Autodesk Inventor part; units mm, degrees
(part 2 of 3)
sketch "CylindricalPathOption2" plane through (0, 0, 0) normal (0, 1, 0) x (1, 0, 0)
  circle A0 centre (-38.1, 345.52) radius 3.175 projected
  circle A1 centre (-88.9, 345.52) radius 3.175 projected
  line L0 (-139.469, 321.04) -> (-139.469, 70.086)
  line L1 (-139.469, 321.04) -> (-144.509, 321.04)
  line L2 (-38.1, 459.82) -> (-101.369, 459.82)
  circle A2 centre (-101.369, 459.82) radius 3.175
  line L3 (-101.369, 459.82) -> (-139.469, 459.82)
  circle A3 centre (-139.469, 459.82) radius 3.175
  line L4 (-139.469, 459.82) -> (-139.469, 357.4623)
  circle A4 centre (-134.429, 321.04) radius 1.016
  line L5 (-139.469, 459.82) -> (-139.469, 321.04)
  line L6 (-139.469, 321.04) -> (-134.429, 321.04)
  circle A5 centre (-139.469, 321.04) radius 3.175
  circle A6 centre (-144.509, 321.04) radius 1.016
  line L7 (-139.469, 459.82) -> (-239.869, 459.82)
  circle A7 centre (-239.869, 459.82) radius 3.175
  circle A8 centre (-134.429, 70.086) radius 1.016
  circle A9 centre (-144.509, 70.086) radius 1.016
  circle A10 centre (-139.469, 70.086) radius 3.175
  line L8 (-139.469, 70.086) -> (-139.469, -143.414)
  circle A11 centre (-134.429, -143.414) radius 1.016
  circle A12 centre (-144.509, -143.414) radius 1.016
  circle A13 centre (-139.469, -143.414) radius 3.175
  line L9 (-38.1, 459.82) -> (-26.0664, 459.82)
  line L10 (-26.0664, 459.82) -> (-26.0664, 471.8536)
  circle A14 centre (-22.5281, 468.3152) radius 1.016
  circle A15 centre (-29.6048, 475.3919) radius 1.016
  circle A16 centre (-26.0664, 471.8536) radius 3.175
  line L11 (-38.1, 459.82) -> (-101.369, 459.82) projected
  point P0 (0, 0)
  point P1 (-38.1, 345.52)
  point P2 (-88.9, 345.52)
  point P3 (-134.429, 70.086)
  dimension "d423" = 12.0335
  dimension "d424" = 12.0335
  dimension "d425" = 6.35
  dimension "d426" = 2.032
  dimension "d427" = 2.032
  dimension "d428" = 63.269
  dimension "d429" = 6.35
  dimension "d430" = 38.1
  dimension "d431" = 100.4
  dimension "d432" = 138.78
  dimension "d433" = 250.954
  dimension "d434" = 213.5
  dimension "d435" = 5.04
  dimension "d436" = 5.04
  dimension "d437" = 2.032
  dimension "d438" = 2.032
  dimension "d439" = 6.35
  dimension "d440" = 5.04
  dimension "d441" = 5.04
  dimension "d442" = 2.032
  dimension "d443" = 2.032
  dimension "d444" = 6.35
  dimension "d445" = 5.04
  dimension "d446" = 5.04
  dimension "d447" = 2.032
  dimension "d448" = 2.032
  dimension "d449" = 6.35
  constraints: 22 end point, 15 centre point, 12 coincident, 2 horizontal, 2 point on line, 1 perpendicular, 1 vertical
  measures "d423" distance of L2.start L9.end
  measures "d424" distance of L9.end L10.end
  measures "d425" diameter of A16
  measures "d426" diameter of A15
  measures "d427" diameter of A14
  measures "d428" distance of L2.start L2.end
  measures "d429" diameter of A2
  measures "d430" distance of L3.start L3.end
  measures "d431" distance of L7.start L7.end
  measures "d432" distance of L5.start L1.start
  measures "d433" distance of L1.start L0.end
  measures "d434" distance of L0.end L8.end
  measures "d435" distance of L1.start L6.end
  measures "d436" distance of L1.start L1.end
  measures "d437" diameter of A6
  measures "d438" diameter of A4
  measures "d439" diameter of A5
  measures "d440" distance of point (-139.469, 70.086) point (-134.429, 70.086)
  measures "d441" distance of point (-139.469, 70.086) point (-144.509, 70.086)
  measures "d442" diameter of A9
  measures "d443" diameter of A8
  measures "d444" diameter of A10
  measures "d445" distance of point (-139.469, -143.414) point (-134.429, -143.414)
  measures "d446" distance of point (-139.469, -143.414) point (-144.509, -143.414)
  measures "d447" diameter of A12
  measures "d448" diameter of A11
  measures "d449" diameter of A13
sketch "CylindricalPathOption3" plane through (0, 0, 0) normal (0, 1, 0) x (1, 0, 0)
  circle A0 centre (-38.1, 80.7174) radius 3.175
  line L0 (-38.1, 320.3874) -> (-43.104, 320.3874)
  line L1 (-38.1, 320.3874) -> (-33.096, 320.3874)
  circle A1 centre (-33.096, 320.3874) radius 1.016
  circle A2 centre (-43.104, 320.3874) radius 1.016
  circle A3 centre (-38.1, 320.3874) radius 3.175
  line L2 (-38.1, 282.2874) -> (-43.104, 282.2874)
  circle A4 centre (-43.104, 282.2874) radius 1.016
  line L3 (-38.1, 282.2874) -> (-38.1, 320.3874)
  line L4 (-38.1, 282.2874) -> (-33.096, 282.2874)
  circle A5 centre (-38.1, 282.2874) radius 3.175
  circle A6 centre (-33.096, 282.2874) radius 1.016
  line L5 (-38.1, 244.1874) -> (-43.104, 244.1874)
  line L6 (-38.1, 244.1874) -> (-33.096, 244.1874)
  circle A7 centre (-33.096, 244.1874) radius 1.016
  circle A8 centre (-43.104, 244.1874) radius 1.016
  circle A9 centre (-38.1, 244.1874) radius 3.175
  line L7 (-38.1, 244.1874) -> (-38.1, 282.2874)
  line L8 (-38.1, 413.5374) -> (-33.096, 413.5374)
  line L9 (-38.1, 413.5374) -> (-38.1, 591.1064)
  circle A10 centre (-33.096, 413.5374) radius 1.016
  circle A11 centre (-33.096, 409.7056) radius 1.016
  circle A12 centre (-33.096, 80.7174) radius 1.016
  circle A13 centre (-43.104, 80.7174) radius 1.016
  circle A14 centre (-38.1, 80.7174) radius 3.175
  line L10 (-38.1, 68.0174) -> (-38.1, 80.7174)
  line L11 (0, 68.0174) -> (-38.1, 68.0174)
  line L12 (-38.1, 80.7174) -> (-33.096, 80.7174)
  line L13 (-38.1, 80.7174) -> (-43.104, 80.7174)
  line L14 (-38.1, 80.7174) -> (-38.1, 156.9174)
  line L15 (-38.1, 156.9174) -> (-43.104, 156.9174)
  line L16 (-38.1, 156.9174) -> (-33.096, 156.9174)
  circle A15 centre (-33.096, 156.9174) radius 1.016
  circle A16 centre (-43.104, 156.9174) radius 1.016
  circle A17 centre (-38.1, 156.9174) radius 3.175
  line L17 (-38.1, 156.9174) -> (-38.1, 174.0274)
  circle A18 centre (-33.096, 174.0274) radius 1.016
  line L18 (-38.1, 174.0274) -> (-33.096, 174.0274)
  line L19 (-38.1, 174.0274) -> (-38.1, 244.1874)
  line L20 (-38.1, 174.0274) -> (-43.104, 174.0274)
  circle A19 centre (-38.1, 174.0274) radius 3.175
  circle A20 centre (-43.104, 174.0274) radius 1.016
  line L21 (-38.1, 320.3874) -> (-38.1, 413.5374)
  line L22 (-38.1, 591.1064) -> (-38.1, 629.2064)
  circle A21 centre (-38.1, 591.1064) radius 3.175
  circle A22 centre (-33.096, 591.1064) radius 1.016
  line L23 (-38.1, 629.2064) -> (-43.104, 629.2064)
  line L24 (-38.1, 629.2064) -> (-33.096, 629.2064)
  circle A23 centre (-33.096, 629.2064) radius 1.016
  circle A24 centre (-43.104, 629.2064) radius 1.016
  circle A25 centre (-38.1, 629.2064) radius 3.175
  line L25 (-38.1, 591.1064) -> (-33.096, 591.1064)
  line L26 (-38.1, 591.1064) -> (-43.104, 591.1064)
  circle A26 centre (-43.104, 591.1064) radius 1.016
  line L27 (-38.1, 413.5374) -> (-38.1, 409.7056)
  circle A27 centre (-38.1, 409.7056) radius 3.175
  circle A28 centre (-38.1, 413.5374) radius 3.175
  line L28 (-38.1, 413.5374) -> (-43.104, 413.5374)
  circle A29 centre (-43.104, 409.7056) radius 1.016
  circle A30 centre (-43.104, 413.5374) radius 1.016
  circle A31 centre (-83.896, 413.5374) radius 1.016
  line L29 (-38.1, 413.5374) -> (-88.9, 413.5374)
  circle A32 centre (-88.9, 413.5374) radius 3.175
  circle A33 centre (-84.547, 90.1756) radius 1.016
  line L30 (-38.1, 629.2064) -> (-38.1, 729.6064)
  line L31 (-38.1, 729.6064) -> (-43.104, 729.6064)
  line L32 (-38.1, 729.6064) -> (-33.096, 729.6064)
  circle A34 centre (-43.104, 729.6064) radius 1.016
  circle A35 centre (-33.096, 729.6064) radius 1.016
  circle A36 centre (-38.1, 729.6064) radius 3.175
  line L33 (-63.5, 742.3174) -> (-38.1, 742.3174)
  line L34 (-38.1, 729.6064) -> (-38.1, 742.3174)
  line L35 (-38.1, 413.5374) -> (-38.1, 451.6374)
  line L36 (-14.6636, 459.2391) -> (108.4085, 459.2391) construction
  line L37 (108.4085, 459.2391) -> (108.4085, 436.8992) construction
  line L38 (108.4085, 436.8992) -> (-14.6636, 436.8992) construction
  line L39 (-14.6636, 436.8992) -> (-14.6636, 459.2391) construction
  line L40 (-38.1, 413.5374) -> (-38.1, 527.8374)
  line L41 (-38.1, 527.8374) -> (-101.369, 527.8374)
  line L42 (-139.469, 527.8374) -> (-239.869, 527.8374)
  circle A37 centre (-239.869, 527.8374) radius 3.175
  circle A38 centre (-139.469, 527.8374) radius 3.175
  circle A39 centre (-101.369, 527.8374) radius 3.175
  line L43 (-101.369, 527.8374) -> (-139.469, 527.8374)
  line L44 (-139.469, 389.0574) -> (-144.509, 389.0574)
  line L45 (-139.469, 527.8374) -> (-139.469, 389.0574)
  circle A40 centre (-144.509, 389.0574) radius 1.016
  line L46 (-139.469, 389.0574) -> (-134.429, 389.0574)
  circle A41 centre (-139.469, 389.0574) radius 3.175
  circle A42 centre (-134.429, 389.0574) radius 1.016
  line L47 (-139.469, 389.0574) -> (-139.469, 138.1034)
  line L48 (-139.469, 527.8374) -> (-139.469, 425.4797)
  circle A43 centre (-139.469, 138.1034) radius 3.175
  circle A44 centre (-144.509, 138.1034) radius 1.016
  circle A45 centre (-134.429, -75.3966) radius 1.016
  line L49 (-139.469, 138.1034) -> (-139.469, -75.3966)
  circle A46 centre (-144.509, -75.3966) radius 1.016
  circle A47 centre (-139.469, -75.3966) radius 3.175
  circle A48 centre (-134.429, 138.1034) radius 1.016
  line L50 (-38.1, 527.8374) -> (-101.369, 527.8374)
  line L51 (-38.1, 527.8374) -> (-26.0664, 527.8374)
  line L52 (-26.0664, 527.8374) -> (-26.0664, 539.871)
  circle A49 centre (-29.6048, 543.4093) radius 1.016
  circle A50 centre (-22.5281, 536.3326) radius 1.016
  circle A51 centre (-26.0664, 539.871) radius 3.175
  circle A52 centre (-26.0664, 539.871) radius 3.175 projected
  circle A53 centre (-29.6048, 543.4093) radius 1.0125 projected
  circle A54 centre (-22.5281, 536.3326) radius 1.0125 projected
  point P0 (0, 0)
  point P1 (0, 68.0174)
  point P2 (-38.1, 409.7056)
  dimension "d450" = 38.1
  dimension "d451" = 12.7
  dimension "d452" = 76.2
  dimension "d453" = 17.11
  dimension "d454" = 70.16
  dimension "d455" = 38.1
  dimension "d456" = 38.1
  dimension "d457" = 93.15
  dimension "d458" = 177.569
  dimension "d459" = 38.1
  dimension "d460" = 100.4
  dimension "d461" = 5.004
  dimension "d462" = 5.004
  dimension "d463" = 2.032
  dimension "d464" = 2.032
  dimension "d465" = 6.35
  dimension "d466" = 5.004
  dimension "d467" = 5.004
  dimension "d468" = 2.032
  dimension "d469" = 2.032
  dimension "d470" = 6.35
  dimension "d471" = 5.004
  dimension "d472" = 5.004
  dimension "d473" = 2.032
  dimension "d474" = 2.032
  dimension "d475" = 6.35
  dimension "d476" = 5.004
  dimension "d477" = 5.004
  dimension "d478" = 2.032
  dimension "d479" = 2.032
  dimension "d480" = 6.35
  dimension "d481" = 5.004
  dimension "d482" = 5.004
  dimension "d483" = 2.032
  dimension "d484" = 2.032
  dimension "d485" = 6.35
  dimension "d486" = 5.004
  dimension "d487" = 5.004
  dimension "d488" = 2.032
  dimension "d489" = 2.032
  dimension "d490" = 6.35
  dimension "d491" = 5.004
  dimension "d492" = 5.004
  dimension "d493" = 2.032
  dimension "d494" = 2.032
  dimension "d495" = 6.35
  dimension "d496" = 5.004
  dimension "d497" = 5.004
  dimension "d498" = 2.032
  dimension "d499" = 2.032
  dimension "d500" = 6.35
  dimension "d501" = 5.004
  dimension "d502" = 5.004
  dimension "d503" = 2.032
  dimension "d504" = 2.032
  dimension "d505" = 6.35
  dimension "d506" = 5.004
  dimension "d507" = 5.004
  dimension "d508" = 2.032
  dimension "d509" = 2.032
  dimension "d510" = 6.35
  dimension "d511" = 50.8
  dimension "d512" = 2.032
  dimension "d513" = 2.032
  constraints: 98 end point, 52 centre point, 42 coincident, 24 horizontal, 11 point on line, 3 vertical, 2 perpendicular, 2 other
  measures "d450" distance of L11.start L10.start
  measures "d451" distance of L10.start L13.start
  measures "d452" distance of L13.start L14.end
  measures "d453" distance of L14.end L19.start
  measures "d454" distance of L19.start L7.start
  measures "d455" distance of L7.start L7.end
  measures "d456" distance of L7.end L3.end
  measures "d457" distance of L3.end L9.start
  measures "d458" distance of L9.start L9.end
  measures "d459" distance of L9.end L22.end
  measures "d460" distance of L22.end L30.end
  measures "d461" distance of L13.start L12.end
  measures "d462" distance of L13.start L13.end
  measures "d463" diameter of A12
  measures "d464" diameter of A13
  measures "d465" diameter of A14
  measures "d466" distance of L15.start L16.end
  measures "d467" distance of L15.start L15.end
  measures "d468" diameter of A15
  measures "d469" diameter of A16
  measures "d470" diameter of A17
  measures "d471" distance of L20.start L18.end
  measures "d472" distance of L20.start L20.end
  measures "d473" diameter of A18
  measures "d474" diameter of A20
  measures "d475" diameter of A19
  measures "d476" distance of L5.start L6.end
  measures "d477" distance of L5.start L5.end
  measures "d478" diameter of A7
  measures "d479" diameter of A8
  measures "d480" diameter of A9
  measures "d481" distance of L2.start L4.end
  measures "d482" distance of L2.start L2.end
  measures "d483" diameter of A6
  measures "d484" diameter of A4
  measures "d485" diameter of A5
  measures "d486" distance of L1.start L1.end
  measures "d487" distance of L1.start L0.end
  measures "d488" diameter of A1
  measures "d489" diameter of A2
  measures "d490" diameter of A3
  measures "d491" distance of L29.start L8.end
  measures "d492" distance of L29.start L28.end
  measures "d493" diameter of A10
  measures "d494" diameter of A30
  measures "d495" diameter of A28
  measures "d496" distance of L26.start L25.end
  measures "d497" distance of L26.start L26.end
  measures "d498" diameter of A22
  measures "d499" diameter of A26
  measures "d500" diameter of A21
  measures "d501" distance of L23.start L24.end
  measures "d502" distance of L23.start L23.end
  measures "d503" diameter of A23
  measures "d504" diameter of A24
  measures "d505" diameter of A25
  measures "d506" distance of L31.start L32.end
  measures "d507" distance of L31.start L31.end
  measures "d508" diameter of A35
  measures "d509" diameter of A34
  measures "d510" diameter of A36
  measures "d511" distance of L29.start L29.end
  measures "d512" diameter of A31
  measures "d513" diameter of A33
sketch "CylindricalPathOption3_CTaslmHoles" plane through (0, 0, 0) normal (0, 1, 0) x (1, 0, 0)
  circle A0 centre (-139.469, 389.0574) radius 3.175 projected
  line L0 (-139.469, 389.0574) -> (-139.469, 156.3064)
  line L1 (-139.469, 156.3064) -> (-139.469, -53.4156)
  circle A1 centre (-144.509, 389.0574) radius 1.016 projected
  line L2 (-139.469, 389.0574) -> (-144.509, 389.0574) projected
  line L3 (-139.469, 389.0574) -> (-134.429, 389.0574) projected
  circle A2 centre (-134.429, 389.0574) radius 1.016 projected
  line L4 (-139.469, 389.0574) -> (-139.469, 138.1034) projected
  line L5 (-139.469, 527.8374) -> (-139.469, 389.0574) projected
  circle A3 centre (-139.469, 156.3064) radius 3.175
  circle A4 centre (-139.469, -53.4156) radius 3.175
  line L6 (-139.469, 156.3064) -> (-144.473, 156.3064)
  line L7 (-139.469, 156.3064) -> (-134.465, 156.3064)
  circle A5 centre (-144.473, 156.3064) radius 1.016
  circle A6 centre (-134.465, 156.3064) radius 1.016
  circle A7 centre (-139.469, -53.4156) radius 3.175
  line L8 (-139.469, -53.4156) -> (-144.473, -53.4156)
  line L9 (-139.469, -53.4156) -> (-134.465, -53.4156)
  circle A8 centre (-144.473, -53.4156) radius 1.016
  circle A9 centre (-134.465, -53.4156) radius 1.016
  circle A10 centre (-139.469, 389.0574) radius 3.175
  line L10 (-139.469, 389.0574) -> (-144.473, 389.0574)
  line L11 (-139.469, 389.0574) -> (-134.465, 389.0574)
  circle A11 centre (-144.473, 389.0574) radius 1.016
  circle A12 centre (-134.465, 389.0574) radius 1.016
  point P0 (0, 0)
  dimension "d549" = 232.751
  dimension "d550" = 209.722
  dimension "d551" = 5.004
  dimension "d552" = 5.004
  dimension "d553" = 2.032
  dimension "d554" = 2.032
  dimension "d555" = 5.004
  dimension "d556" = 5.004
  dimension "d557" = 2.032
  dimension "d558" = 2.032
  dimension "d559" = 5.004
  dimension "d560" = 5.004
  dimension "d561" = 2.032
  dimension "d562" = 2.032
  constraints: 16 end point, 10 centre point, 8 coincident, 6 horizontal, 1 point on line, 1 vertical
  measures "d549" distance of L0.start L0.end
  measures "d550" distance of L0.end L1.end
  measures "d551" distance of L6.start L7.end
  measures "d552" distance of L6.start L6.end
  measures "d553" diameter of A5
  measures "d554" diameter of A6
  measures "d555" distance of L8.start L9.end
  measures "d556" distance of L8.start L8.end
  measures "d557" diameter of A8
  measures "d558" diameter of A9
  measures "d559" distance of L10.start L11.end
  measures "d560" distance of L10.start L10.end
  measures "d561" diameter of A11
  measures "d562" diameter of A12
sketch "CYlindricalPathOption3_VCHoles" plane through (0, 0, 0) normal (0, 1, 0) x (1, 0, 0)
  line L0 (-239.869, 527.8374) -> (-262.099, 527.8374)
  line L1 (-262.099, 527.8374) -> (-338.999, 527.8374)
  line L2 (-338.999, 527.8374) -> (-341.695, 527.8374)
  line L3 (-303.8023, 535.3668) -> (-291.2854, 535.3668) construction
  line L4 (-291.2854, 535.3668) -> (-291.2854, 507.3746) construction
  line L5 (-291.2854, 507.3746) -> (-303.8023, 507.3746) construction
  line L6 (-303.8023, 507.3746) -> (-303.8023, 535.3668) construction
  line L7 (-254.611, 288.2795) -> (478.2477, 288.2795) construction
  line L8 (478.2477, 288.2795) -> (478.2477, 269.1629) construction
  line L9 (463.9102, 269.1629) -> (463.9102, 514.9312) construction
  line L10 (-343.8716, 547.7163) -> (-320.6585, 547.7163) construction
  line L11 (-320.6585, 547.7163) -> (-320.6585, 536.5649) construction
  line L12 (-320.6585, 536.5649) -> (-343.8716, 536.5649) construction
  line L13 (-343.8716, 536.5649) -> (-343.8716, 547.7163) construction
  line L14 (-341.695, 527.8374) -> (-346.521, 527.8374)
  line L15 (-350.0636, 516.5149) -> (379.7144, 289.8633) construction
  line L16 (379.7144, 289.8633) -> (-315.8667, 507.5645) construction
  line L17 (-330.3348, 498.5727) -> (-350.0636, 516.5149) construction
  line L18 (-346.521, 527.8374) -> (-384.621, 527.8374)
  line L19 (-384.621, 527.8374) -> (-435.421, 527.8374)
  line L20 (-369.5637, 503.4304) -> (-369.5637, 514.5818) construction
  line L21 (-369.5637, 514.5818) -> (-346.3506, 514.5818) construction
  line L22 (-346.3506, 514.5818) -> (-346.3506, 503.4304) construction
  line L23 (-346.3506, 503.4304) -> (-369.5637, 503.4304) construction
  line L24 (-384.621, 527.8374) -> (-384.621, 502.4374)
  line L25 (-384.621, 527.8374) -> (-384.621, 553.2374)
  line L26 (-435.421, 527.8374) -> (-435.421, 502.4374)
  line L27 (-435.421, 527.8374) -> (-450.661, 527.8374)
  circle A0 centre (-239.869, 527.8374) radius 3.175 projected
  line L28 (-412.024, 603.0828) -> (-94.0009, 603.0828) construction
  line L29 (-94.0009, 603.0828) -> (-94.0009, 575.0095) construction
  line L30 (-94.0009, 575.0095) -> (-412.024, 575.0095) construction
  line L31 (-412.024, 575.0095) -> (-412.024, 603.0828) construction
  point P0 (0, 0)
  point P1 (-254.611, 514.9312)
  dimension "d563" = 22.23
  dimension "d564" = 76.9
  dimension "d565" = 2.696
  dimension "d566" = 4.826
  dimension "d567" = 38.1
  dimension "d568" = 50.8
  dimension "d569" = 25.4
  dimension "d570" = 25.4
  dimension "d571" = 25.4
  dimension "d572" = 15.24
  constraints: 20 end point, 4 horizontal, 3 point on line, 3 vertical, 10 other
  measures "d563" distance of L0.start L1.start
  measures "d564" distance of L1.start L1.end
  measures "d565" distance of L1.end L14.start
  measures "d566" distance of L14.start L14.end
  measures "d567" distance of L14.end L18.end
  measures "d568" distance of L18.end L19.end
  measures "d569" distance of L18.end L24.end
  measures "d570" distance of L18.end L25.end
  measures "d571" distance of L19.end L26.end
  measures "d572" distance of L19.end L27.end
hole "Hole2" [suppressed]
sketch "Sketch16" plane through (0, 0, 0) normal (0, 1, 0) x (1, 0, 0)
  circle A0 centre (-139.469, -75.3966) radius 3.175 projected
  line L0 (-139.469, -75.3966) -> (-101.369, -75.3966)
  line L1 (-101.369, -75.3966) -> (-101.369, -88.0966)
  line L2 (-101.369, -88.0966) -> (-177.569, -88.0966)
  line L3 (-127, 489.7374) -> (-127, 0) projected
  line L4 (-127, 0) -> (0, 0) projected
  line L5 (-310.6166, 489.7374) -> (-127, 489.7374) projected
  line L6 (-177.569, -88.0966) -> (-177.569, 489.7374)
  line L7 (-101.369, -75.3966) -> (-101.369, 0)
  dimension "d580" = 38.1
  dimension "d581" = 12.7
  dimension "d582" = 76.2
  constraints: 10 end point, 2 horizontal, 2 perpendicular, 2 point on line, 1 vertical
  measures "d580" distance of L0.start L0.end
  measures "d581" distance of L0.end L1.end
  measures "d582" distance of L1.end L2.end
extrude "Extrusion12" [suppressed]
sketch "CylindricalPathOption4" plane through (0, 0, 0) normal (0, 1, 0) x (1, 0, 0)
  line L0 (-204.8612, 436.8992) -> (-204.8612, 459.2391) construction
  line L1 (-204.8612, 459.2391) -> (-81.7891, 459.2391) construction
  line L2 (-81.7891, 459.2391) -> (-81.7891, 436.8992) construction
  line L3 (-81.7891, 436.8992) -> (-204.8612, 436.8992) construction
  circle A0 centre (-223.2936, 413.5374) radius 1.0125
  line L4 (-228.2976, 413.5374) -> (-228.2976, 451.6374)
  line L5 (-228.2976, 413.5374) -> (-228.2976, 527.8374)
  line L6 (-228.2976, 413.5374) -> (-228.2976, 591.1064)
  circle A1 centre (-233.3016, 413.5374) radius 1.0125
  circle A2 centre (-228.2976, 413.5374) radius 3.175
  line L7 (-228.2976, 413.5374) -> (-279.0976, 413.5374)
  circle A3 centre (-274.0936, 413.5374) radius 1.0125
  circle A4 centre (-279.0976, 413.5374) radius 3.175
  line L8 (-228.2976, 591.1064) -> (-233.3016, 591.1064)
  circle A5 centre (-233.3016, 591.1064) radius 1.0125
  circle A6 centre (-228.2976, 591.1064) radius 3.175
  line L9 (-228.2976, 591.1064) -> (-223.2936, 591.1064)
  circle A7 centre (-223.2936, 591.1064) radius 1.0125
  line L10 (-228.2976, 591.1064) -> (-228.2976, 629.2064)
  line L11 (-228.2976, 629.2064) -> (-233.3016, 629.2064)
  line L12 (-228.2976, 629.2064) -> (-223.2936, 629.2064)
  circle A8 centre (-233.3016, 629.2064) radius 1.0125
  circle A9 centre (-223.2936, 629.2064) radius 1.0125
  circle A10 centre (-228.2976, 629.2064) radius 3.175
  line L13 (-228.2976, 527.8374) -> (-291.5666, 527.8374)
  line L14 (-228.2976, 282.2874) -> (-233.3016, 282.2874)
  line L15 (-228.2976, 282.2874) -> (-223.2936, 282.2874)
  circle A11 centre (-233.3016, 244.1874) radius 1.0125
  line L16 (-228.2976, 244.1874) -> (-233.3016, 244.1874)
  circle A12 centre (-228.2976, 244.1874) radius 3.175
  line L17 (-228.2976, 244.1874) -> (-228.2976, 282.2874)
  line L18 (-228.2976, 244.1874) -> (-223.2936, 244.1874)
  circle A13 centre (-223.2936, 244.1874) radius 1.0125
  line L19 (-228.2976, 156.9174) -> (-233.3016, 156.9174)
  line L20 (-228.2976, 156.9174) -> (-223.2936, 156.9174)
  circle A14 centre (-223.2936, 156.9174) radius 1.0125
  circle A15 centre (-233.3016, 156.9174) radius 1.0125
  circle A16 centre (-228.2976, 156.9174) radius 3.175
  line L21 (-228.2976, 80.7174) -> (-233.3016, 80.7174)
  circle A17 centre (-233.3016, 80.7174) radius 1.0125
  circle A18 centre (-228.2976, 80.7174) radius 3.175
  circle A19 centre (-228.2976, 80.7174) radius 3.175
  line L22 (-228.2976, 80.7174) -> (-228.2976, 156.9174)
  circle A20 centre (-223.2936, 80.7174) radius 1.0125
  circle A21 centre (-274.7446, 90.1756) radius 1.0125
  circle A22 centre (-223.2936, 282.2874) radius 1.0125
  circle A23 centre (-228.2976, 282.2874) radius 3.175
  line L23 (-228.2976, 320.3874) -> (-223.2936, 320.3874)
  line L24 (-228.2976, 282.2874) -> (-228.2976, 320.3874)
  line L25 (-228.2976, 320.3874) -> (-233.3016, 320.3874)
  circle A24 centre (-223.2936, 320.3874) radius 1.0125
  circle A25 centre (-233.3016, 320.3874) radius 1.0125
  circle A26 centre (-228.2976, 320.3874) radius 3.175
  circle A27 centre (-233.3016, 282.2874) radius 1.0125
  line L26 (-228.2976, 174.0274) -> (-228.2976, 244.1874)
  line L27 (-228.2976, 174.0274) -> (-233.3016, 174.0274)
  circle A28 centre (-233.3016, 174.0274) radius 1.0125
  circle A29 centre (-223.2936, 174.0274) radius 1.0125
  circle A30 centre (-228.2976, 174.0274) radius 3.175
  line L28 (-228.2976, 156.9174) -> (-228.2976, 174.0274)
  line L29 (-228.2976, 174.0274) -> (-223.2936, 174.0274)
  line L30 (-228.2976, 68.0174) -> (-228.2976, 80.7174)
  line L31 (-190.1976, 68.0174) -> (-228.2976, 68.0174)
  line L32 (-228.2976, 80.7174) -> (-223.2936, 80.7174)
  line L33 (-228.2976, 413.5374) -> (-223.2936, 413.5374)
  circle A31 centre (-223.2936, 409.7056) radius 1.0125
  line L34 (-228.2976, 320.3874) -> (-228.2976, 413.5374)
  circle A32 centre (-233.3016, 409.7056) radius 1.0125
  circle A33 centre (-228.2976, 409.7056) radius 3.175
  line L35 (-228.2976, 413.5374) -> (-233.3016, 413.5374)
  line L36 (-228.2976, 413.5374) -> (-228.2976, 409.7056)
  line L37 (-228.2976, 629.2064) -> (-228.2976, 729.6064)
  line L38 (-228.2976, 729.6064) -> (-233.3016, 729.6064)
  line L39 (-228.2976, 729.6064) -> (-223.2936, 729.6064)
  circle A34 centre (-223.2936, 729.6064) radius 1.0125
  circle A35 centre (-233.3016, 729.6064) radius 1.0125
  circle A36 centre (-228.2976, 729.6064) radius 3.175
  line L40 (-253.6976, 742.3174) -> (-228.2976, 742.3174)
  line L41 (-228.2976, 729.6064) -> (-228.2976, 742.3174)
  line L42 (-291.5666, 527.8374) -> (-329.6666, 527.8374)
  circle A37 centre (-329.6666, 527.8374) radius 3.175
  circle A38 centre (-430.0666, 527.8374) radius 3.175
  line L43 (-329.6666, 527.8374) -> (-430.0666, 527.8374)
  circle A39 centre (-291.5666, 527.8374) radius 3.175
  line L44 (-228.2976, 527.8374) -> (-291.5666, 527.8374)
  line L45 (-228.2976, 527.8374) -> (-216.264, 527.8374)
  line L46 (-216.264, 527.8374) -> (-216.264, 539.871)
  circle A40 centre (-212.7257, 536.3326) radius 1.0125
  circle A41 centre (-219.8024, 543.4093) radius 1.0125
  circle A42 centre (-216.264, 539.871) radius 3.175
  circle A43 centre (-329.6666, 527.8374) radius 3.175 projected
  line L47 (-329.6666, 527.8374) -> (-348.7166, 527.8374)
  line L48 (-348.7166, 389.0574) -> (-348.7166, 138.1034)
  circle A44 centre (-348.7166, 389.0574) radius 3.175
  circle A45 centre (-348.7166, -75.3966) radius 3.175
  line L49 (-348.7166, 138.1034) -> (-348.7166, -75.3966)
  circle A46 centre (-348.7166, 138.1034) radius 3.175
  line L50 (-348.7166, 527.8374) -> (-348.7166, 425.4797)
  line L51 (-348.7166, 527.8374) -> (-348.7166, 389.0574)
  circle A47 centre (-266.1666, 532.8414) radius 1.0125 projected
  circle A48 centre (-266.1666, 522.8334) radius 1.0125 projected
  circle A49 centre (-266.1666, 527.8374) radius 3.175 projected
  line L52 (-291.5666, 527.8374) -> (-291.5666, 522.8334)
  line L53 (-291.5666, 522.8334) -> (-291.5666, 532.8414)
  line L54 (-430.0666, 527.8374) -> (-430.0666, 522.8334)
  line L55 (-430.0666, 522.8334) -> (-430.0666, 532.8414)
  circle A50 centre (-291.5666, 532.8414) radius 1.0125
  circle A51 centre (-291.5666, 522.8334) radius 1.0125
  circle A52 centre (-430.0666, 532.8414) radius 1.0125
  circle A53 centre (-430.0666, 522.8334) radius 1.0125
  line L56 (-279.0976, 413.5374) -> (-284.1016, 413.5374)
  circle A54 centre (-284.1016, 413.5374) radius 1.0125
  line L57 (-348.7166, 389.0574) -> (-353.7206, 389.0574)
  circle A55 centre (-348.7166, 379.0684) radius 3.175 projected
  circle A56 centre (-343.7126, 379.0684) radius 1.0125 projected
  circle A57 centre (-353.7206, 379.0684) radius 1.0125 projected
  line L58 (-353.7206, 379.0684) -> (-353.7206, 389.0574)
  line L59 (-348.7166, 138.1034) -> (-353.7206, 138.1034)
  line L60 (-348.7166, 138.1034) -> (-343.7126, 138.1034)
  line L61 (-348.7166, -75.3966) -> (-353.7206, -75.3966)
  line L62 (-348.7166, -75.3966) -> (-343.7126, -75.3966)
  line L63 (-291.5666, 527.8374) -> (-291.5666, 522.8334)
  circle A58 centre (-353.7206, 389.0574) radius 1.0125
  circle A59 centre (-343.7126, 138.1034) radius 1.0125
  circle A60 centre (-353.7206, 138.1034) radius 1.0125
  circle A61 centre (-343.7126, -75.3966) radius 1.0125
  circle A62 centre (-353.7206, -75.3966) radius 1.0125
  line L64 (-348.7166, 389.0574) -> (-343.7126, 389.0574)
  circle A63 centre (-343.7126, 389.0574) radius 1.0125
  point P0 (0, 0)
  point P1 (-190.1976, 68.0174)
  point P2 (-228.2976, 409.7056)
  point P3 (-353.7566, 138.1034)
  dimension "d585" = 38.1
  dimension "d586" = 12.7
  dimension "d587" = 76.2
  dimension "d588" = 17.11
  dimension "d589" = 70.16
  dimension "d590" = 38.1
  dimension "d591" = 38.1
  dimension "d592" = 93.15
  dimension "d593" = 177.569
  dimension "d594" = 38.1
  dimension "d595" = 100.4
  dimension "d596" = 5.004
  dimension "d597" = 5.004
  dimension "d598" = 2.025
  dimension "d599" = 2.025
  dimension "d600" = 6.35
  dimension "d601" = 5.004
  dimension "d602" = 5.004
  dimension "d603" = 2.025
  dimension "d604" = 2.025
  dimension "d605" = 6.35
  dimension "d606" = 5.004
  dimension "d607" = 5.004
  dimension "d608" = 2.025
  dimension "d609" = 2.025
  dimension "d610" = 6.35
  dimension "d611" = 5.004
  dimension "d612" = 5.004
  dimension "d613" = 2.025
  dimension "d614" = 2.025
  dimension "d615" = 6.35
  dimension "d616" = 5.004
  dimension "d617" = 5.004
  dimension "d618" = 2.025
  dimension "d619" = 2.025
  dimension "d620" = 6.35
  dimension "d621" = 5.004
  dimension "d622" = 5.004
  dimension "d623" = 2.025
  dimension "d624" = 2.025
  dimension "d625" = 6.35
  dimension "d626" = 5.004
  dimension "d627" = 5.004
  dimension "d628" = 2.025
  dimension "d629" = 2.025
  dimension "d630" = 6.35
  dimension "d631" = 5.004
  dimension "d632" = 5.004
  dimension "d633" = 2.025
  dimension "d634" = 2.025
  dimension "d635" = 6.35
  dimension "d636" = 5.004
  dimension "d637" = 5.004
  dimension "d638" = 2.025
  dimension "d639" = 2.025
  dimension "d640" = 6.35
  dimension "d641" = 5.004
  dimension "d642" = 5.004
  dimension "d643" = 2.025
  dimension "d644" = 2.025
  dimension "d645" = 6.35
  dimension "d646" = 50.8
  dimension "d647" = 2.025
  dimension "d648" = 2.025
  constraints: 122 end point, 57 centre point, 47 coincident, 29 horizontal, 14 point on line, 6 vertical, 2 perpendicular, 1 collinear, 2 other
  measures "d585" distance of L31.start L30.start
  measures "d586" distance of L30.start L21.start
  measures "d587" distance of L21.start L28.start
  measures "d588" distance of L28.start L26.start
  measures "d589" distance of L26.start L17.start
  measures "d590" distance of L17.start L17.end
  measures "d591" distance of L17.end L34.start
  measures "d592" distance of L34.start L6.start
  measures "d593" distance of L6.start L6.end
  measures "d594" distance of L6.end L37.start
  measures "d595" distance of L37.start L37.end
  measures "d596" distance of L21.start L32.end
  measures "d597" distance of L21.start L21.end
  measures "d598" diameter of A20
  measures "d599" diameter of A17
  measures "d600" diameter of A19
  measures "d601" distance of L20.start L20.end
  measures "d602" distance of L20.start L19.end
  measures "d603" diameter of A14
  measures "d604" diameter of A15
  measures "d605" diameter of A16
  measures "d606" distance of L27.start L29.end
  measures "d607" distance of L27.start L27.end
  measures "d608" diameter of A29
  measures "d609" diameter of A28
  measures "d610" diameter of A30
  measures "d611" distance of L16.start L18.end
  measures "d612" distance of L16.start L16.end
  measures "d613" diameter of A13
  measures "d614" diameter of A11
  measures "d615" diameter of A12
  measures "d616" distance of L14.start L15.end
  measures "d617" distance of L14.start L14.end
  measures "d618" diameter of A22
  measures "d619" diameter of A27
  measures "d620" diameter of A23
  measures "d621" distance of L25.start L23.end
  measures "d622" distance of L25.start L25.end
  measures "d623" diameter of A24
  measures "d624" diameter of A25
  measures "d625" diameter of A26
  measures "d626" distance of L7.start L33.end
  measures "d627" distance of L7.start L35.end
  measures "d628" diameter of A0
  measures "d629" diameter of A1
  measures "d630" diameter of A2
  measures "d631" distance of L8.start L9.end
  measures "d632" distance of L8.start L8.end
  measures "d633" diameter of A7
  measures "d634" diameter of A5
  measures "d635" diameter of A6
  measures "d636" distance of L11.start L12.end
  measures "d637" distance of L11.start L11.end
  measures "d638" diameter of A9
  measures "d639" diameter of A8
  measures "d640" diameter of A10
  measures "d641" distance of L39.start L39.end
  measures "d642" distance of L39.start L38.end
  measures "d643" diameter of A34
  measures "d644" diameter of A35
  measures "d645" diameter of A36
  measures "d646" distance of L7.start L7.end
  measures "d647" diameter of A3
  measures "d648" diameter of A21
sketch "CylindricalPathOption4_VCHoles" plane through (0, 0, 0) normal (0, 1, 0) x (1, 0, 0)
  line L0 (-510.8561, 536.5649) -> (-534.0692, 536.5649) construction
  line L1 (-510.8561, 547.7163) -> (-510.8561, 536.5649) construction
  line L2 (-452.2966, 527.8374) -> (-529.1966, 527.8374)
  line L3 (-430.0666, 527.8374) -> (-452.2966, 527.8374)
  line L4 (-534.0692, 547.7163) -> (-510.8561, 547.7163) construction
  line L5 (-516.8401, 591.9265) -> (826.1994, 174.8104) construction
  line L6 (-531.8926, 527.8374) -> (-536.7186, 527.8374)
  line L7 (-534.0692, 536.5649) -> (-534.0692, 547.7163) construction
  line L8 (-529.1966, 527.8374) -> (-531.8926, 527.8374)
  line L9 (-493.9999, 535.3668) -> (-481.483, 535.3668) construction
  line L10 (-493.9999, 507.3746) -> (-493.9999, 535.3668) construction
  line L11 (-481.483, 535.3668) -> (-481.483, 507.3746) construction
  line L12 (-444.8086, 173.2266) -> (924.7328, 173.2266) construction
  line L13 (-481.483, 507.3746) -> (-493.9999, 507.3746) construction
  line L14 (910.3953, 154.11) -> (910.3953, 514.9312) construction
  line L15 (822.8003, 163.9498) -> (92.5183, 392.5116) construction
  line L16 (116.1502, 383.5198) -> (-309.3135, 770.4574) construction
  line L17 (-536.7186, 527.8374) -> (-574.8186, 527.8374)
  line L18 (-559.7613, 514.5818) -> (-536.5482, 514.5818) construction
  line L19 (-574.8186, 527.8374) -> (-574.8186, 553.2374)
  line L20 (-559.7613, 503.4304) -> (-559.7613, 514.5818) construction
  line L21 (-536.5482, 514.5818) -> (-536.5482, 503.4304) construction
  line L22 (-536.5482, 503.4304) -> (-559.7613, 503.4304) construction
  line L23 (-574.8186, 527.8374) -> (-574.8186, 502.4374)
  line L24 (-574.8186, 527.8374) -> (-625.6186, 527.8374)
  line L25 (-625.6186, 527.8374) -> (-625.6186, 502.4374)
  line L26 (-625.6186, 527.8374) -> (-640.8586, 527.8374)
  line L27 (-602.2216, 575.0095) -> (-602.2216, 603.0828) construction
  line L28 (-602.2216, 603.0828) -> (-284.1985, 603.0828) construction
  line L29 (-284.1985, 603.0828) -> (-284.1985, 575.0095) construction
  line L30 (-284.1985, 575.0095) -> (-602.2216, 575.0095) construction
  circle A0 centre (-430.0666, 527.8374) radius 3.175 projected
  point P0 (0, 0)
  point P1 (-540.2612, 516.5149)
  point P2 (-444.8086, 514.9312)
  point P3 (826.1994, 174.8104)
  point P4 (92.5183, 392.5116)
  point P5 (116.1502, 383.5198)
  dimension "d684" = 22.23
  dimension "d685" = 76.9
  dimension "d686" = 2.696
  dimension "d687" = 4.826
  dimension "d688" = 38.1
  dimension "d689" = 50.8
  dimension "d690" = 25.4
  dimension "d691" = 25.4
  dimension "d692" = 25.4
  dimension "d693" = 15.24
  constraints: 20 end point, 4 horizontal, 3 point on line, 3 vertical, 10 other
  measures "d684" distance of L3.start L2.start
  measures "d685" distance of L2.start L8.start
  measures "d686" distance of L8.start L8.end
  measures "d687" distance of L8.end L6.end
  measures "d688" distance of L6.end L17.end
  measures "d689" distance of L17.end L25.start
  measures "d690" distance of L17.end L23.end
  measures "d691" distance of L17.end L19.end
  measures "d692" distance of L25.start L25.end
  measures "d693" distance of L25.start L26.end
hole "Hole3" at (-574.8186, 0, -502.4374) at (-574.8186, 0, -553.2374) at (-625.6186, 0, -502.4374) direction (0, -1, 0) diameter 4.9784 end through all thread size "1/4-20 UNC" class "2B" standard "ANSI Unified Screw Threads"
sketch "CylindricalPathOption4_CTaslmHoles" plane through (0, 0, 0) normal (0, 1, 0) x (1, 0, 0)
  line L0 (-348.7166, 389.0574) -> (-348.7166, 156.3064)
  line L1 (-348.7166, 156.3064) -> (-348.7166, -53.4156)
  circle A0 centre (-348.7166, 156.3064) radius 3.175
  circle A1 centre (-348.7166, -53.4156) radius 3.175
  line L2 (-348.7166, 156.3064) -> (-353.7206, 156.3064)
  line L3 (-348.7166, 156.3064) -> (-343.7126, 156.3064)
  circle A2 centre (-353.7206, 156.3064) radius 1.0125
  circle A3 centre (-343.7126, 156.3064) radius 1.0125
  circle A4 centre (-353.7206, -53.4156) radius 1.0125
  line L4 (-348.7166, -53.4156) -> (-353.7206, -53.4156)
  circle A5 centre (-348.7166, -53.4156) radius 3.175
  line L5 (-348.7166, -53.4156) -> (-343.7126, -53.4156)
  circle A6 centre (-343.7126, -53.4156) radius 1.0125
  circle A7 centre (-353.7206, 389.0574) radius 1.0125
  line L6 (-348.7166, 389.0574) -> (-353.7206, 389.0574)
  circle A8 centre (-348.7166, 389.0574) radius 3.175
  line L7 (-348.7166, 389.0574) -> (-343.7126, 389.0574)
  circle A9 centre (-343.7126, 389.0574) radius 1.0125
  circle A10 centre (-348.7166, 389.0574) radius 3.175 projected
  point P0 (0, 0)
  point P1 (-348.7166, 138.1034)
  dimension "d720" = 232.751
  dimension "d721" = 209.722
  dimension "d722" = 5.004
  dimension "d723" = 5.004
  dimension "d724" = 2.025
  dimension "d725" = 2.025
  dimension "d726" = 5.004
  dimension "d727" = 5.004
  dimension "d728" = 2.025
  dimension "d729" = 2.025
  dimension "d730" = 5.004
  dimension "d731" = 5.004
  dimension "d732" = 2.025
  dimension "d733" = 2.025
  constraints: 16 end point, 10 centre point, 8 coincident, 6 horizontal, 1 point on line, 1 vertical
  measures "d720" distance of L0.start L1.start
  measures "d721" distance of L1.start L1.end
  measures "d722" distance of L3.start L3.end
  measures "d723" distance of L3.start L2.end
  measures "d724" diameter of A2
  measures "d725" diameter of A3
  measures "d726" distance of L5.start L5.end
  measures "d727" distance of L5.start L4.end
  measures "d728" diameter of A4
  measures "d729" diameter of A6
  measures "d730" distance of L6.start L7.end
  measures "d731" distance of L6.start L6.end
  measures "d732" diameter of A7
  measures "d733" diameter of A9
sketch "Sketch20" plane through (0, 0, 0) normal (0, 1, 0) x (1, 0, 0)
  line L0 (-310.6166, 489.7374) -> (-127, 489.7374) projected
  line L1 (-310.6166, -59.2176) -> (-310.6166, 489.7374) projected
  line L2 (-127, 489.7374) -> (-127, 0) projected
  line L3 (-127, 0) -> (-310.6166, 0)
  point P0 (0, 0)
  constraints: 2 end point, 1 perpendicular, 1 point on line
extrude "Extrusion13" add sketch "Sketch20" against normal blind 12.7
move faces "Move1" translate (-12.7, 0, 0) faces at (-310.6166, -4.2333, 39.4784) (-244.3361, -12.7, -256.2606)
move faces "Move2" translate (12.7, 0, 0) faces at (-386.8166, -8.4667, -306.7524)
move faces "Move3" translate (0, 0, 25.4) faces at (-357.1833, -4.2333, 59.2176)
extrude "CPO4_InnerHolesASLM" cut sketch "CylindricalPathOption4" against normal blind 12.7 contours A33 A2 L34 | L34 A2 A33 | A2 L34 A33 | A33 L34 A2 | A4 L56 L7 | L7 L56 A4 | A39 L52 L13 | L13 L53 A39 | L52 A39 L42 | L42 A39 L53 | L17 A23 L14 | L24 A23 L15 | L15 A23 L17 | L14 A23 L24 | L26 A12 L16 | L16 A12 L17 | L17 A12 L18 | L18 A12 L26 | L22 A16 L19 | L28 A16 L20 | L20 A16 L22 | L19 A16 L28 | L30 A18 L21 | L21 A18 L22 | L32 A18 L30 | L22 A18 L32 | L34 A26 L23 | L23 A26 L24 | L24 A26 L25 | L25 A26 L34 | L27 A30 L26 | L28 A30 L27 | L29 A30 L28 | L26 A30 L29 | L43 L55 A38 | A38 L54 L43 | L55 L54 A38 | A42 | L64 A44 L48 | L57 A44 L51 | L48 A44 L57 | L51 A44 L64 | A46 L60 L48 | L48 L59 A46 | L60 A46 L49 | L49 A46 L59 | L62 L49 A45 | A45 L61 L62 | L49 L61 A45
extrude "CPO4_InnerHolesCTASLM" cut sketch "CylindricalPathOption4_CTaslmHoles" against normal blind 12.7 contours A0 L3 L0 | L0 L2 A0 | L3 A0 L1 | L1 A0 L2 | A1 L5 L1 | L1 L4 A1 | L5 A1 L4
sketch "MountHolesOuter_CylindricalOption4" plane through (-705.4595, -12.7, -565.9374) normal (0, -1, 0) x (1, 0, 0)
  arc A0 (358.9221, 617.0439) -> (354.5638, 617.0439) centre (356.7429, 619.353) ccw projected
  arc A1 (354.5638, 617.0439) -> (358.9221, 617.0439) centre (356.7429, 612.455) ccw projected
  circle A2 centre (356.7429, 409.631) radius 3.175 projected
  arc A3 (358.0943, 424.961) -> (355.3916, 424.961) centre (356.7429, 427.834) ccw projected
  arc A4 (355.3916, 424.961) -> (358.0943, 424.961) centre (356.7429, 420.064) ccw projected
  circle A5 centre (477.1619, 391.91) radius 3.175 projected
  circle A6 centre (477.1619, 156.2318) radius 3.175 projected
  circle A7 centre (275.3929, 38.1) radius 3.175 projected
  circle A8 centre (356.7429, 641.334) radius 3.175 projected
  circle A9 centre (413.8929, 38.1) radius 3.175 projected
  circle A10 centre (477.1619, 245.55) radius 3.175 projected
  circle A11 centre (477.1619, 409.02) radius 3.175 projected
  circle A12 centre (477.1619, 321.75) radius 3.175 projected
  circle A13 centre (426.3619, 152.4) radius 3.175 projected
  circle A14 centre (356.7429, 176.88) radius 3.175 projected
  circle A15 centre (489.1955, 26.0664) radius 3.175 projected
  circle A16 centre (477.1619, 283.65) radius 3.175 projected
  circle A17 centre (477.1619, 485.22) radius 3.175 projected
  circle A18 centre (79.8409, 63.5) radius 2.4892 projected
  circle A19 centre (130.6409, 12.7) radius 2.4892 projected
  circle A20 centre (130.6409, 63.5) radius 2.4892 projected
  circle A21 centre (356.7429, 438.255) radius 5.08 projected
  circle A22 centre (667.3595, 227.0174) radius 5.08 projected
  circle A23 centre (667.3595, 409.0924) radius 5.08 projected
  circle A24 centre (679.3931, 26.0664) radius 5.08 projected
  circle A25 centre (274.326, 50.1336) radius 5.08 projected
  circle A26 centre (286.3595, 12.7) radius 5.08 projected
  circle A27 centre (667.3595, 392.2014) radius 5.08 projected
  circle A28 centre (375.7929, 38.1) radius 5.08 projected
  circle A29 centre (356.7429, 599.964) radius 5.08 projected
  circle A30 centre (667.3595, 553.2374) radius 5.08 projected
  circle A31 centre (667.3595, 322.0974) radius 5.08 projected
  circle A32 centre (616.5595, 76.2) radius 5.08 projected
  circle A33 centre (210.792, 38.1) radius 5.08 projected
  circle A34 centre (439.2929, 38.1) radius 5.08 projected
  circle A35 centre (667.3595, 141.6558) radius 5.08 projected
  circle A36 centre (667.3595, 489.7374) radius 5.08 projected
  circle A37 centre (356.7429, 186.869) radius 5.08 projected
  circle A38 centre (362.5595, 70.6374) radius 3.175 projected
  circle A39 centre (591.1595, 553.2374) radius 3.175 projected
  circle A40 centre (692.7595, 19.8374) radius 3.175 projected
  circle A41 centre (6.9595, 70.6374) radius 3.175 projected
  circle A42 centre (692.7595, 553.2374) radius 3.175 projected
  circle A43 centre (591.1595, 70.6374) radius 3.175 projected
  circle A44 centre (6.9595, 19.8374) radius 3.175 projected
  circle A45 centre (362.5595, 578.6374) radius 3.175 projected
  circle A46 centre (66.04, 12.7) radius 2.4892 projected
  circle A47 centre (15.24, 63.5) radius 2.4892 projected
  circle A48 centre (66.04, 63.5) radius 2.4892 projected
  line L0 (705.4595, 565.9374) -> (382.1429, 565.9374) projected
  line L1 (382.1429, 565.9374) -> (382.1429, 650.555) projected
  line L2 (382.1429, 650.555) -> (331.3429, 650.555) projected
  line L3 (331.3429, 650.555) -> (331.3429, 76.2) projected
  line L4 (331.3429, 76.2) -> (0, 76.2) projected
  line L5 (0, 76.2) -> (0, 0) projected
  line L6 (0, 0) -> (705.4595, 0) projected
  line L7 (705.4595, 0) -> (705.4595, 565.9374) projected
  circle A49 centre (477.1619, 485.22) radius 5.08
  circle A50 centre (477.1619, 409.02) radius 5.08
  circle A51 centre (477.1619, 391.91) radius 5.08
  circle A52 centre (477.1619, 321.75) radius 5.08
  circle A53 centre (477.1619, 283.65) radius 5.08
  circle A54 centre (477.1619, 245.55) radius 5.08
  circle A55 centre (477.1619, 156.2318) radius 5.08
  circle A56 centre (413.8929, 38.1) radius 5.08
  circle A57 centre (275.3929, 38.1) radius 5.08
  circle A58 centre (426.3619, 152.4) radius 5.08
  circle A59 centre (356.7429, 176.88) radius 5.08
  circle A60 centre (356.7429, 409.631) radius 5.08
  circle A61 centre (356.7429, 427.834) radius 5.08
  circle A62 centre (356.7429, 619.353) radius 5.08
  circle A63 centre (356.7429, 641.334) radius 5.08
  circle A64 centre (489.1955, 26.0664) radius 5.08
  dimension "d749" = 10.16
  dimension "d750" = 10.16
  dimension "d751" = 10.16
  dimension "d752" = 10.16
  dimension "d753" = 10.16
  dimension "d754" = 10.16
  dimension "d755" = 10.16
  dimension "d756" = 10.16
  dimension "d757" = 10.16
  dimension "d758" = 10.16
  dimension "d759" = 10.16
  dimension "d760" = 10.16
  dimension "d761" = 10.16
  dimension "d762" = 10.16
  dimension "d763" = 10.16
  dimension "d764" = 10.16
  constraints: 16 centre point, 1 coincident
  measures "d749" diameter of A49
  measures "d750" diameter of A50
  measures "d751" diameter of A51
  measures "d752" diameter of A52
  measures "d753" diameter of A53
  measures "d754" diameter of A54
  measures "d755" diameter of A55
  measures "d756" diameter of A56
  measures "d757" diameter of A57
  measures "d758" diameter of A58
  measures "d759" diameter of A59
  measures "d760" diameter of A60
  measures "d761" diameter of A61
  measures "d762" diameter of A62
  measures "d763" diameter of A63
  measures "d764" diameter of A64
extrude "CPO4_OuterHoles" cut sketch "MountHolesOuter_CylindricalOption4" against normal blind 7.62 contours A1 A62 A0 | A0 A1 A62 | A2 | A4 A61 A3 | A3 A4 A61 | A5 | A6 | A7 | A8 | A9 | A10 | A11 | A12 | A13 | A14 | A15 | A16 | A17 | A59 A37 | A37 A59 | A49 | A50 | A51 | A52 | A53 | A54 | A55 | A56 | A57 | A58 | A60 | A63 | A64 picked at (356.8465, 181.8492) picked at (361.14, 176.4802)
extrude "CPO4_DowellPinsASLM" cut sketch "CylindricalPathOption4" against normal blind 4.445 contours A3 L7 | L7 A3 | A11 | A13 | A14 | A15 | A17 | A20 | A22 | A24 | A25 | A27 | A28 | A29 | A31 | A32 | A40 | A41 | A50 | A51 | A52 | A53 | A54 | A58 L58 L57 | L57 L58 A58 | A59 | A60 | A61 | A62 | A63
extrude "CPO4_DowelPinsCTASLM" cut sketch "CylindricalPathOption4_CTaslmHoles" against normal blind 4.445 contours A2 | A3 | A4 | A6 | A7
sketch "Sketch22" plane through (0, 0, 0) normal (0, 1, 0) x (1, 0, 0)
  circle A0 centre (-348.7166, 389.0574) radius 3.175 projected
  circle A1 centre (-329.6666, 527.8374) radius 3.175 projected
  line L0 (-329.6666, 527.8374) -> (-348.7166, 527.8374)
  line L1 (-348.7166, 527.8374) -> (-348.7166, 591.3374)
  circle A2 centre (-348.7166, 591.3374) radius 3.175
  arc A3 (-352.7081, 389.0574) -> (-352.7081, 389.0574) centre (-353.7566, 389.0574) ccw projected
  arc A4 (-352.7081, 389.0574) -> (-352.7081, 389.0574) centre (-353.7206, 389.0574) ccw projected
  circle A5 centre (-343.7126, 379.0684) radius 1.0125 projected
  circle A6 centre (-353.7206, 379.0684) radius 1.0125 projected
  line L2 (-348.7166, 591.3374) -> (-353.7206, 591.3374)
  line L3 (-348.7166, 591.3374) -> (-343.7126, 591.3374)
  circle A7 centre (-343.7126, 591.3374) radius 1.0125
  circle A8 centre (-353.7206, 591.3374) radius 1.0125
  line L4 (-348.7166, 591.3374) -> (-348.7166, 604.0374)
  line L5 (-348.7166, 604.0374) -> (-329.6666, 604.0374)
  line L6 (-348.7166, 604.0374) -> (-367.7666, 604.0374)
  line L7 (0, 565.9374) -> (-705.4595, 565.9374) projected
  line L8 (-367.7666, 604.0374) -> (-329.6666, 604.0374)
  line L9 (-329.6666, 604.0374) -> (-329.6666, 565.9374)
  line L10 (-329.6666, 565.9374) -> (-367.7666, 565.9374)
  line L11 (-367.7666, 565.9374) -> (-367.7666, 604.0374)
  point P0 (0, 0)
  dimension "d777" = 63.5
  dimension "d778" = 5.004
  dimension "d779" = 5.004
  dimension "d793" = 2.025
  dimension "d794" = 2.025
  dimension "d795" = 12.7
  dimension "d796" = 19.05
  dimension "d797" = 19.05
  constraints: 22 end point, 5 horizontal, 3 centre point, 3 coincident, 2 parallel, 2 perpendicular, 2 vertical, 1 point on line, 1 other
  measures "d777" distance of L0.end L1.end
  measures "d778" distance of L2.start L2.end
  measures "d779" distance of L2.start L3.end
  measures "d793" diameter of A7
  measures "d794" diameter of A8
  measures "d795" distance of L2.start L4.end
  measures "d796" distance of L4.end L5.end
  measures "d797" distance of L4.end L6.end
extrude "Extrusion19" add sketch "Sketch22" against normal blind 12.7 contours L7 L11 L6 L4 A2 L1 | L1 A2 L4 L5 L9 L7 | A2 L2 L1 | L1 L3 A2 | L4 A2 L3 | L2 A2 L4 | A7 | A8
extrude "Extrusion20" cut sketch "Sketch22" against normal blind 4.445 contours A7 | A8
extrude "Extrusion21" cut sketch "Sketch22" against normal blind 25.4 contours A2 L2 L1 | L1 L3 A2 | L4 A2 L3 | L2 A2 L4
sketch "Sketch23" plane through (-323.3166, -12.7, 0) normal (0, -1, 0) x (1, 0, 0)
  circle A0 centre (-25.4, -591.3374) radius 3.175 projected
  circle A1 centre (-95.7834, -553.2374) radius 5.08 projected
  circle A2 centre (-25.4, -591.3374) radius 5.08
  point P0 (323.3166, 0)
  dimension "d804" = 10.16
  constraints: 1 centre point, 1 coincident
  measures "d804" diameter of A2
extrude "Extrusion22" cut sketch "Sketch23" against normal blind 7.62 contours A0 | A2
sketch "Sketch24" plane through (0, 0, 0) normal (0, 1, 0) x (1, 0, 0)
  line L0 (-686.5286, 294.8704) -> (-395.8685, 294.8704) construction
  line L1 (-395.8685, 294.8704) -> (-395.8685, 13.5864) construction
  line L2 (-395.8685, 13.5864) -> (-686.5286, 13.5864) construction
  line L3 (-686.5286, 13.5864) -> (-686.5286, 294.8704) construction
  point P0 (0, 0)
  constraints: 2 other